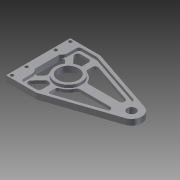
# Autodesk Inventor part: lower bix side plate 3
Saved by Autodesk Inventor 2012 (Build 160160000, 160)
## iProperties
Created: 2012-12-28
Part Number: lower bix side plate 3
Material: Default
Document SubType Name: Modeling
Designer: Bryce
Density: 1 g/cm^3
Author: Bryce
Autodesk Inventor part; units mm, degrees
ref_plane "YZ Plane" through (0, 0, 0) normal (1, 0, 0) x (0, 1, 0)
ref_plane "XZ Plane" through (0, 0, 0) normal (0, 1, 0) x (-1, 0, 0)
ref_plane "XY Plane" through (0, 0, 0) normal (0, 0, 1) x (1, 0, 0)
sketch "Sketch1" plane through (0, 0, 0) normal (0, 0, 1) x (1, 0, 0)
  line L0 (-34.925, 101.6) -> (34.925, 101.6)
  line L1 (34.925, 101.6) -> (34.925, 68.8594)
  line L2 (-34.925, 68.8594) -> (-34.925, 101.6)
  line L3 (-34.925, 68.8594) -> (-10.5309, -3.5479)
  line L4 (34.925, 68.8594) -> (10.5309, -3.5479)
  arc A0 (-10.5309, -3.5479) -> (10.5309, -3.5479) centre (0, 0) ccw
  circle A1 centre (0, 0) radius 4.7625
  circle A2 centre (0, 68.8594) radius 11.1125
  line L5 (0, 68.8594) -> (-34.925, 68.8594) construction
  line L6 (0, 68.8594) -> (34.925, 68.8594) construction
  line L7 (0, 68.8594) -> (-34.925, 101.6) construction
  line L8 (0, 68.8594) -> (34.925, 101.6) construction
  line L9 (0, 68.8594) -> (0, 0) construction
  line L10 (0, 68.8594) -> (0, 0) construction
  arc A3 (-15.5543, 65.6844) -> (-4.7625, 53.7156) centre (0, 68.8594) ccw
  arc A4 (4.7625, 53.7156) -> (15.5543, 65.6844) centre (0, 68.8594) ccw
  arc A5 (15.5543, 72.0344) -> (13.5191, 77.181) centre (0, 68.8594) ccw
  arc A6 (9.1762, 81.8137) -> (-9.1762, 81.8137) centre (0, 68.8594) ccw
  arc A7 (-13.5191, 77.181) -> (-15.5543, 72.0344) centre (0, 68.8594) ccw
  line L11 (-4.7625, 53.7156) -> (-4.7625, 10.0402)
  line L12 (4.7625, 53.7156) -> (4.7625, 10.0402)
  arc A8 (-4.7625, 10.0402) -> (-7.7188, 7.9942) centre (0, 0) ccw
  arc A9 (7.7188, 7.9942) -> (4.7625, 10.0402) centre (0, 0) ccw
  line L13 (-27.1547, 65.6844) -> (-7.7188, 7.9942)
  line L14 (7.7188, 7.9942) -> (27.1547, 65.6844)
  line L15 (-27.1547, 65.6844) -> (-15.5543, 65.6844)
  line L16 (-28.575, 72.0344) -> (-15.5543, 72.0344)
  line L17 (15.5543, 65.6844) -> (27.1547, 65.6844)
  line L18 (15.5543, 72.0344) -> (28.575, 72.0344)
  line L19 (-28.575, 91.2952) -> (-13.5191, 77.181)
  line L20 (-20.1222, 92.075) -> (-9.1762, 81.8137)
  line L21 (20.1222, 92.075) -> (9.1762, 81.8137)
  line L22 (28.575, 91.2952) -> (13.5191, 77.181)
  line L23 (-28.575, 91.2952) -> (-28.575, 72.0344)
  line L24 (-20.1222, 92.075) -> (20.1222, 92.075)
  line L25 (28.575, 91.2952) -> (28.575, 72.0344)
  arc A10 (4.7625, 18.588) -> (10.9463, 17.5744) centre (7.9375, 18.588) ccw
  arc A11 (-10.9463, 17.5744) -> (-4.7625, 18.588) centre (-7.9375, 18.588) ccw
  point P0 (-31.75, 98.425)
  point P1 (31.75, 98.425)
  point P2 (-15.875, 98.425)
  point P3 (15.875, 98.425)
  dimension "d0" = 69.85
  dimension "d1" = 101.6
  dimension "d2" = 34.925
  dimension "d6" = 18.619
  dimension "d7" = 9.525
  dimension "d8" = 32.7406
  dimension "d9" = 22.225
  dimension "d12" = 15.875
  dimension "d13" = 4.7625
  dimension "d14" = 4.7625
  dimension "d15" = 6.35
  dimension "d16" = 6.35
  dimension "d17" = 3.175
  dimension "d18" = 3.175
  dimension "d19" = 3.175
  dimension "d20" = 3.175
  dimension "d21" = 3.175
  dimension "d22" = 3.175
  dimension "d24" = 3.175
  dimension "d25" = 3.175
  dimension "d26" = 6.35
  dimension "d27" = 9.525
  dimension "d28" = 6.35
  dimension "d32" = 3.175
  dimension "d33" = 3.175
  dimension "d35" = 3.175
  dimension "d36" = 3.175
  dimension "d62" = 19.05
  dimension "d63" = 19.05
  dimension "d69" = 3.175
  dimension "d70" = 18.619
  dimension "d71" = 11.1125
  constraints: 52 end point, 20 point on circle, 13 parallel, 12 centre point, 9 coincident, 7 equal radius, 7 perpendicular, 5 tangent, 4 horizontal alignment, 4 point on line, 1 collinear, 1 horizontal, 1 vertical alignment
  measures "d0" distance between parallel lines of L1 L2
  measures "d1" distance from line of point (0, 0) L0
  measures "d2" distance from line of point (0, 0) L2
  measures "d6" angle of L1 L4
  measures "d7" diameter of A1
  measures "d8" distance from line of L5.start L0
  measures "d9" diameter of A2
  measures "d12" radius of A3
  measures "d13" distance between parallel lines of L9 L11
  measures "d14" distance between parallel lines of L9 L12
  measures "d15" distance between parallel lines of L3 L13
  measures "d16" distance between parallel lines of L4 L14
  measures "d17" distance between parallel lines of L15 L5
  measures "d18" distance between parallel lines of L5 L16
  measures "d19" distance between parallel lines of L17 L6
  measures "d20" distance between parallel lines of L6 L18
  measures "d21" distance between parallel lines of L8 L21
  measures "d22" distance between parallel lines of L8 L22
  measures "d24" distance between parallel lines of L7 L19
  measures "d25" distance between parallel lines of L7 L20
  measures "d26" distance between parallel lines of L23 L2
  measures "d27" distance between parallel lines of L0 L24
  measures "d28" distance between parallel lines of L1 L25
  measures "d32" distance from line of L2 point (-31.75, 98.425)
  measures "d33" distance from line of L0 point (-31.75, 98.425)
  measures "d35" distance from line of L0 point (31.75, 98.425)
  measures "d36" distance from line of L1 point (31.75, 98.425)
  measures "d62" distance from line of L2 point (-15.875, 98.425)
  measures "d63" distance from line of point (15.875, 98.425) L1
  measures "d69" radius of A11
  measures "d70" angle of L3 L2
  measures "d71" radius of A0
extrude "Extrusion1" add sketch "Sketch1" against normal blind 3.175 contours L0 L1 L4 A0 L3 L2 | A3 L11 A11 L13 L15 | L11 A8 L13 A11 | A4 L17 L14 A10 L12 | A10 L14 A9 L12 | A5 L22 L25 L18 | A6 L20 L24 L21 | A7 L16 L23 L19
extrude "Extrusion2" cut sketch "Sketch1" against normal blind 3.175 contours A3 L11 A11 L13 L15 | A4 L17 L14 A10 L12 | A5 L22 L25 L18 | A6 L20 L24 L21 | A7 L16 L23 L19
fillet "Fillet1" radius 3.175 16 edges at (-28.575, 72.0344, -1.5875) (-28.575, 91.2952, -1.5875) (28.575, 91.2952, -1.5875) (28.575, 72.0344, -1.5875) (15.5543, 72.0344, -1.5875) (13.5191, 77.181, -1.5875) (9.1762, 81.8137, -1.5875) (-9.1762, 81.8137, -1.5875) (-13.5191, 77.181, -1.5875) (-15.5543, 72.0344, -1.5875) (15.5543, 65.6844, -1.5875) (27.1547, 65.6844, -1.5875) (4.7625, 53.7156, -1.5875) (-4.7625, 53.7156, -1.5875) (-15.5543, 65.6844, -1.5875) (-27.1547, 65.6844, -1.5875)
hole "Hole1" at (-31.75, 98.425, 0) at (31.75, 98.425, 0) at (-15.875, 98.425, 0) at (15.875, 98.425, 0) direction (0, 0, -1) diameter 3.6576 end through all
sketch "Sketch2" plane through (0, 0, 0) normal (0, 0, 1) x (1, 0, 0)
  circle A0 centre (31.75, 98.425) radius 1.8288 projected
  circle A1 centre (-31.75, 98.425) radius 1.8288 projected
  line L0 (20.1222, 92.075) -> (10.9317, 83.4593) projected
  arc A2 (7.3002, 82.9563) -> (10.9317, 83.4593) centre (8.7602, 85.7757) ccw projected
  arc A3 (7.3002, 82.9563) -> (-7.3002, 82.9563) centre (0, 68.8594) ccw projected
  arc A4 (-10.9317, 83.4593) -> (-7.3002, 82.9563) centre (-8.7602, 85.7757) ccw projected
  line L1 (-10.9317, 83.4593) -> (-20.1222, 92.075) projected
  line L2 (-20.1222, 92.075) -> (20.1222, 92.075) projected
  circle A5 centre (0, 68.8594) radius 11.1125 projected
  circle A6 centre (0, 0) radius 4.7625 projected
  line L3 (-34.925, 68.8594) -> (-34.925, 101.6) projected
  line L4 (-10.5309, -3.5479) -> (-34.925, 68.8594) projected
  arc A7 (-10.5309, -3.5479) -> (10.5309, -3.5479) centre (0, 0) ccw projected
  line L5 (34.925, 68.8594) -> (10.5309, -3.5479) projected
  line L6 (34.925, 101.6) -> (34.925, 68.8594) projected
  line L7 (-34.925, 101.6) -> (34.925, 101.6)
  line L8 (34.925, 101.6) -> (34.925, 88.9)
  line L9 (34.925, 88.9) -> (31.75, 88.9) construction
  line L10 (-34.925, 88.9) -> (-34.925, 101.6)
  line L11 (-16.7353, 88.9) -> (-31.75, 88.9)
  line L12 (16.7353, 88.9) -> (-16.7353, 88.9) construction
  line L13 (-31.75, 88.9) -> (-31.75, 69.3799)
  line L14 (-31.75, 69.3799) -> (-10.0051, 4.8359)
  line L15 (31.75, 88.9) -> (31.75, 69.3799)
  line L16 (31.75, 69.3799) -> (10.0051, 4.8359)
  arc A8 (0, 11.1125) -> (-10.0051, 4.8359) centre (0, 0) ccw
  arc A9 (10.0051, 4.8359) -> (0, 11.1125) centre (0, 0) ccw
  line L17 (0, 68.8594) -> (0, 0) construction
  line L18 (-31.75, 88.9) -> (-34.925, 88.9) construction
  line L19 (31.75, 88.9) -> (16.7353, 88.9)
  circle A10 centre (15.875, 98.425) radius 1.8288 projected
  circle A11 centre (-15.875, 98.425) radius 1.8288 projected
  circle A12 centre (-15.875, 98.425) radius 1.8288
  circle A13 centre (15.875, 98.425) radius 1.8288
  arc A14 (-14.5384, 75.2352) -> (-14.9671, 74.1511) centre (0, 68.8594) ccw projected
  circle A15 centre (0, 68.8594) radius 14.2875
  dimension "d45" = 12.7
  dimension "d46" = 3.175
  dimension "d47" = 3.175
  dimension "d48" = 3.175
  dimension "d49" = 3.175
  dimension "d53" = 22.225
  dimension "d72" = 28.575
  constraints: 26 end point, 9 parallel, 6 coincident, 5 centre point, 4 concentric, 4 point on circle, 4 point on line, 2 perpendicular, 1 horizontal
  measures "d45" distance between parallel lines of L9 L7
  measures "d46" distance between parallel lines of L3 L13
  measures "d47" distance between parallel lines of L4 L14
  measures "d48" distance between parallel lines of L5 L16
  measures "d49" distance between parallel lines of L6 L15
  measures "d53" diameter of A5
  measures "d72" diameter of A15
extrude "Extrusion4" add sketch "Sketch2" along normal blind 3.175
fillet "Fillet6" radius 3.175 8 edges at (-20.1222, 92.075, 0) (-31.75, 88.9, 1.5875) (-31.75, 69.3799, 1.5875) (31.75, 88.9, 1.5875) (20.1222, 92.075, 0) (31.75, 69.3799, 1.5875) (-10.0051, 4.8359, 1.5875) (10.0051, 4.8359, 1.5875)
fillet "Fillet7" radius 6.35 2 edges at (15.268, 88.9, 1.5875) (-15.268, 88.9, 1.5875)
body "Solid1"
